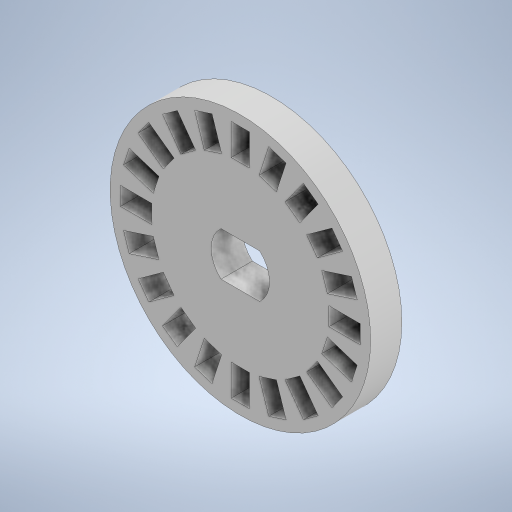
# Autodesk Inventor part: Disco_encoder
Saved by Autodesk Inventor 2023 (Build 270158000, 158)
## iProperties
Created: 2023-06-07
Part Number: Disco_encoder
Material: Genérico
Document SubType Name: Modeling
Designer: sergi
Density: 1 g/cm^3
Appearance: Valor por defecto
Author: sergi
Autodesk Inventor part; units mm, degrees
ref_plane "YZ Plane" through (0, 0, 0) normal (1, 0, 0) x (0, 1, 0)
ref_plane "XZ Plane" through (0, 0, 0) normal (0, 1, 0) x (-1, 0, 0)
ref_plane "XY Plane" through (0, 0, 0) normal (0, 0, 1) x (1, 0, 0)
sketch "Boceto1" plane through (0, 0, 0) normal (0, 0, 1) x (1, 0, 0)
  circle A0 centre (0, 0) radius 12.5
  circle A1 centre (0, 0) radius 2.8
  line L0 (-1.852, 2.1) -> (1.852, 2.1)
  line L1 (-1.852, -2.1) -> (1.852, -2.1)
  dimension "d0" = 25
  dimension "d1" = 5.6
  dimension "d2" = 2.1
  dimension "d3" = 2.1
  constraints: 4 end point, 4 point on circle, 2 centre point, 2 coincident, 1 horizontal
  measures "d0" diameter of A0
  measures "d1" diameter of A1
  measures "d2" distance from line of L0 point (0, 0)
  measures "d3" distance from line of point (0, 0) L1
extrude "Extrusión1" add sketch "Boceto1" along normal blind 3 contours A0 | L0 A1 | A1 L1
sketch "Boceto2" plane through (0, 0, 3) normal (0, 0, 1) x (1, 0, 0)
  line L0 (-0.875, 11.5) -> (0.875, 11.5)
  line L1 (0.875, 11.5) -> (0.875, 8.5)
  line L2 (0.875, 8.5) -> (-0.875, 8.5)
  line L3 (-0.875, 8.5) -> (-0.875, 11.5)
  point P0 (0, 0)
  point P1 (0, 11.5)
  dimension "d6" = 3
  dimension "d7" = 1.75
  dimension "d8" = 8.5
  constraints: 8 end point, 2 parallel, 1 horizontal, 1 midpoint, 1 perpendicular, 1 vertical alignment
  measures "d6" distance of L0.end L1.end
  measures "d7" distance of L0.start L0.end
  measures "d8" distance from line of point (0, 0) L2
extrude "Extrusión2" cut sketch "Boceto2" against normal through all
pattern_circular "Patrón circular1" count 20 over 360 about axis through (0, 0, -10) along (0, 0, 1) of "Extrusión2"
